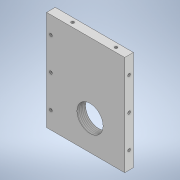
# Autodesk Inventor part: left
Saved by Autodesk Inventor 2022.2 (Build 262287030, 287C)
## iProperties
Created: 2022-01-28
Part Number: left
Material: Generic
Document SubType Name: Modeling
Designer: Tapendra
Density: 1 g/cm^3
Appearance: Default
Author: Tapendra
Autodesk Inventor part; units mm, degrees
ref_plane "YZ Plane" through (0, 0, 0) normal (1, 0, 0) x (0, 1, 0)
ref_plane "XZ Plane" through (0, 0, 0) normal (0, 1, 0) x (-1, 0, 0)
ref_plane "XY Plane" through (0, 0, 0) normal (0, 0, 1) x (1, 0, 0)
sketch "Sketch1" plane through (0, 0, 0) normal (0, 0, 1) x (1, 0, 0)
  line L0 (-45, 57.5) -> (45, 57.5)
  line L1 (45, 57.5) -> (45, -57.5)
  line L2 (45, -57.5) -> (-45, -57.5)
  line L3 (-45, -57.5) -> (-45, 57.5)
  line L4 (-45, 57.5) -> (45, -57.5) construction
  line L5 (45, 57.5) -> (-45, -57.5) construction
  point P0 (0, 0)
  dimension "d0" = 90
  dimension "d1" = 115
  constraints: 12 end point, 2 midpoint, 2 parallel, 1 horizontal, 1 perpendicular
  measures "d0" distance of L0.start L0.end
  measures "d1" distance of L0.end L1.end
extrude "Extrusion1" add sketch "Sketch1" along normal mid plane 10
sketch "Sketch2" plane through (45, -57.5, 5) normal (1, 0, 0) x (0, 0, -1)
  line L0 (10, 0) -> (0, 0) projected
  line L1 (10, 115) -> (10, 0) projected
  point P0 (5, 57.5)
  point P1 (5, 20)
  point P2 (5, 57.5)
  point P3 (5, 95)
  dimension "d4" = 20
  dimension "d5" = 5
  dimension "d8" = 37.5
  constraints: 1 vertical, 2 other
  measures "d4" distance from line of L0 point (5, 20)
  measures "d5" distance from line of L1 point (5, 20)
  measures "d8" distance of point (5, 20) point (5, 57.5)
hole "Hole1" at (45, -37.5, 0) at (45, 0, 0) at (45, 37.5, 0) direction (-1, 0, 0) diameter 3.175 depth 5
sketch "Sketch3" plane through (-45, -57.5, 5) normal (0, -1, 0) x (1, 0, 0)
  line L0 (0, 0) -> (0, -10) projected
  line L1 (90, -10) -> (0, -10) projected
  point P0 (45, -5)
  point P1 (25, -5)
  point P2 (75, -5)
  dimension "d20" = 25
  dimension "d21" = 5
  dimension "d24" = 50
  constraints: 1 horizontal, 1 other
  measures "d20" distance from line of L0 point (25, -5)
  measures "d21" distance from line of L1 point (25, -5)
  measures "d24" distance of point (25, -5) point (75, -5)
hole "Hole2" at (-20, -57.5, 0) at (30, -57.5, 0) direction (0, 1, 0) diameter 3.175 depth 5
sketch "Sketch4" plane through (-45, 57.5, 5) normal (0, 1, 0) x (1, 0, 0)
  line L0 (0, 10) -> (0, 0) projected
  line L1 (90, 0) -> (0, 0) projected
  point P0 (45, 5)
  point P1 (25, 5)
  point P2 (75, 5)
  dimension "d36" = 25
  dimension "d37" = 5
  dimension "d40" = 50
  constraints: 1 horizontal, 1 other
  measures "d36" distance from line of L0 point (25, 5)
  measures "d37" distance from line of L1 point (25, 5)
  measures "d40" distance of point (25, 5) point (75, 5)
hole "Hole3" at (-20, 57.5, 0) at (30, 57.5, 0) direction (0, -1, 0) diameter 3.175 depth 5
sketch "Sketch5" plane through (0, 0, 5) normal (0, 0, 1) x (1, 0, 0)
  line L0 (-45, 57.5) -> (-45, -57.5) projected
  line L1 (-45, -57.5) -> (45, -57.5) projected
  point P0 (0, 0)
  point P1 (-40, -37.5)
  point P2 (-40, 0)
  point P3 (-40, 37.5)
  dimension "d52" = 5
  dimension "d53" = 20
  dimension "d56" = 37.5
  constraints: 1 vertical, 2 other
  measures "d52" distance from line of L0 point (-40, -37.5)
  measures "d53" distance from line of L1 point (-40, -37.5)
  measures "d56" distance of point (-40, -37.5) point (-40, 0)
hole "Hole4" at (-40, -37.5, 5) at (-40, 0, 5) at (-40, 37.5, 5) direction (0, 0, -1) diameter 3.175 depth 5
sketch "Sketch7" plane through (0, 0, -5) normal (0, 0, -1) x (-1, 0, 0)
  circle A0 centre (-5, -23.36) radius 15.085
  line L0 (-45, -57.5) -> (45, -57.5) projected
  line L1 (-45, 57.5) -> (-45, -57.5) projected
  point P0 (0, 0)
  dimension "d74" = 34.14
  dimension "d75" = 40
  dimension "d76" = 30.17
  constraints: 1 centre point
  measures "d74" distance from line of L0 A0.centre
  measures "d75" distance from line of L1 A0.centre
  measures "d76" diameter of A0
extrude "Extrusion3" cut sketch "Sketch7" against normal through all
thread "Thread1" size "3/4" designation "3/4 - 14 NPT" standard "NPT" length 20.15
body "Solid1"
